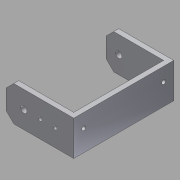
# Autodesk Inventor part: face
Saved by Autodesk Inventor 2014 (Build 180170000, 170)
## iProperties
Created: 2014-10-04
Part Number: face
Material: 一般
Document SubType Name: Modeling
Designer: kayako
Density: 1 g/cm^3
Appearance: 滑らか - 白
Author: kayako
Autodesk Inventor part; units mm, degrees
ref_plane "YZ Plane" through (0, 0, 0) normal (1, 0, 0) x (0, 1, 0)
ref_plane "XZ Plane" through (0, 0, 0) normal (0, 1, 0) x (-1, 0, 0)
ref_plane "XY Plane" through (0, 0, 0) normal (0, 0, 1) x (1, 0, 0)
sketch "スケッチ1" plane through (0, 0, 0) normal (0, 0, 1) x (1, 0, 0)
  line L0 (-20, 7) -> (20, 7)
  line L1 (20, 7) -> (20, -7)
  line L2 (20, -7) -> (-20, -7)
  line L3 (-20, -7) -> (-20, 7)
  line L4 (-28, 0) -> (28, 0) construction
  line L5 (0, -9.8) -> (0, 9.8) construction
  point P0 (0, 0)
  dimension "d0" = 40
  dimension "d1" = 14
  dimension "d2" = 20
  dimension "d3" = 7
  constraints: 8 end point, 2 parallel, 1 horizontal, 1 perpendicular
  measures "d0" distance of L1.end L2.end
  measures "d1" distance of L0.end L1.end
  measures "d2" distance between parallel lines of L3 L5
  measures "d3" distance between parallel lines of L0 L4
extrude "押し出し1" add sketch "スケッチ1" along normal blind 2
sketch "スケッチ2" plane through (0, 0, 2) normal (0, 0, 1) x (1, 0, 0)
  line L0 (-20, -7) -> (20, -7) projected
  line L1 (-20, 7) -> (-18, 7)
  line L2 (-18, 7) -> (-18, -7)
  line L3 (-18, -7) -> (-20, -7)
  line L4 (-20, -7) -> (-20, 7)
  point P0 (0, 0)
  dimension "d6" = 2
  constraints: 8 end point, 2 parallel, 1 horizontal, 1 perpendicular, 1 point on line
  measures "d6" distance of L2.end L3.end
extrude "押し出し2" add sketch "スケッチ2" along normal blind 23
sketch "スケッチ3" plane through (0, 0, 2) normal (0, 0, 1) x (1, 0, 0)
  line L0 (-18, -7) -> (20, -7) projected
  line L1 (20, 7) -> (18, 7)
  line L2 (18, 7) -> (18, -7)
  line L3 (18, -7) -> (20, -7)
  line L4 (20, -7) -> (20, 7)
  point P0 (0, 0)
  dimension "d9" = 2
  constraints: 8 end point, 2 parallel, 1 horizontal, 1 perpendicular, 1 point on line
  measures "d9" distance of L3.end L2.end
extrude "押し出し3" add sketch "スケッチ3" along normal blind 25
sketch "スケッチ4" plane through (20, -7, 0) normal (1, 0, 0) x (0, 0, -1)
  line L0 (-27, 0) -> (-27, 14) projected
  circle A0 centre (-20, 7) radius 1.25
  point P0 (0, 7)
  dimension "d12" = 2.5
  dimension "d13" = 7
  constraints: 1 centre point
  measures "d12" diameter of A0
  measures "d13" distance from line of A0.centre L0
extrude "押し出し4" cut sketch "スケッチ4" against normal blind 27
sketch "スケッチ5" plane through (20, -7, 0) normal (1, 0, 0) x (0, 0, -1)
  circle A0 centre (-20, 7) radius 1.25 projected
  circle A1 centre (-13.5, 7) radius 0.8
  point P0 (0, 7)
  dimension "d16" = 1.6
  dimension "d17" = 6.5
  constraints: 1 centre point
  measures "d16" diameter of A1
  measures "d17" distance of A1.centre A0.centre
extrude "押し出し5" cut sketch "スケッチ5" against normal blind 27 contours A1
sketch "スケッチ6" plane through (20, -7, 0) normal (1, 0, 0) x (0, 0, -1)
  circle A0 centre (-20, 7) radius 1.25 projected
  circle A1 centre (-7.5, 7) radius 0.8
  point P0 (0, 7)
  dimension "d20" = 1.6
  dimension "d21" = 12.5
  constraints: 1 centre point
  measures "d20" diameter of A1
  measures "d21" distance of A0.centre A1.centre
extrude "押し出し6" cut sketch "スケッチ6" against normal blind 27 contours A1
sketch "スケッチ7" plane through (-20, -7, 0) normal (-1, 0, 0) x (0, 0, 1)
  circle A0 centre (20, 7) radius 1.25 projected
  circle A1 centre (20, 7) radius 1.25
  point P0 (0, 7)
  dimension "d24" = 2.5
  constraints: 1 centre point, 1 coincident
  measures "d24" diameter of A1
extrude "押し出し7" cut sketch "スケッチ7" against normal blind 27
sketch "スケッチ8" plane through (0, 0, 2) normal (0, 0, 1) x (1, 0, 0)
  circle A0 centre (-16, 1.5) radius 0.8
  line L0 (-18, -7) -> (18, -7) projected
  line L1 (0, -9.8) -> (0, 9.8) construction
  line L2 (-20, 7) -> (-20, -7) projected
  point P0 (0, 0)
  dimension "d27" = 1.6
  dimension "d37" = 8.5
  dimension "d39" = 4
  constraints: 1 centre point
  measures "d27" diameter of A0
  measures "d37" distance from line of L0 A0.centre
  measures "d39" distance from line of L2 A0.centre
extrude "押し出し8" cut sketch "スケッチ8" against normal blind 27
mirror "ミラー1" about plane through (0, 0, 0) normal (1, 0, 0) of "押し出し8"
chamfer "面取り1" [suppressed]
chamfer "面取り2" distance 3 angle 45 4 edges at (-19, -7, 25) (-19, 7, 25) (19, 7, 27) (19, -7, 27)
sketch "スケッチ9" plane through (0, 0, 0) normal (0, 0, -1) x (-1, 0, 0)
  line L0 (-20, -7) -> (20, -7) projected
  point P0 (0, 0)
  point P1 (-17, 1)
  dimension "d40" = 8
  dimension "d41" = 17
  measures "d40" distance from line of point (-17, 1) L0
  measures "d41" horizontal distance of point (-17, 1) point (0, 0)
equation "\"d2\" = 0.5 * d0"
equation "\"d3\" = 0.5 * d1"
